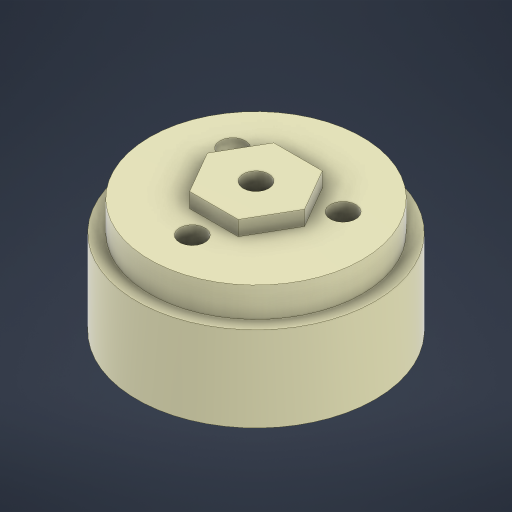
# Autodesk Inventor part: Shaft1_Joint1
Saved by Autodesk Inventor 2023 (Build 270158000, 158)
## iProperties
Created: 2023-02-21
Part Number: Shaft1_Joint1
Material: ABS Plastic
Document SubType Name: Modeling
Designer: dzw04
Density: 1.06 g/cm^3
Appearance: Smooth - Ash
Author: dzw04
Autodesk Inventor part; units mm, degrees
ref_plane "YZ Plane" through (0, 0, 0) normal (1, 0, 0) x (0, 1, 0)
ref_plane "XZ Plane" through (0, 0, 0) normal (0, 1, 0) x (-1, 0, 0)
ref_plane "XY Plane" through (0, 0, 0) normal (0, 0, 1) x (1, 0, 0)
sketch "Sketch1" plane through (0, 0, 0) normal (0, 1, 0) x (-1, 0, 0)
  circle A0 centre (0, 0) radius 14
  dimension "d0" = 28
  constraints: 1 centre point, 1 coincident
  measures "d0" diameter of A0
extrude "Extrusion1" add sketch "Sketch1" along normal blind 10
sketch "Sketch2" plane through (0, 10, 0) normal (0, 1, 0) x (1, 0, 0)
  circle A0 centre (0, 0) radius 12.5
  dimension "d3" = 25
  constraints: 1 centre point, 1 coincident
  measures "d3" diameter of A0
extrude "Extrusion2" add sketch "Sketch2" along normal blind 3.5
sketch "Sketch3" plane through (0, 0, 0) normal (0, -1, 0) x (1, 0, 0)
  circle A0 centre (0, 0) radius 7.5 construction
  circle A1 centre (0, 0) radius 1.5
  circle A2 centre (0, 7.5) radius 1.5
  circle A3 centre (-6.4952, 3.75) radius 1.5
  circle A4 centre (-6.4952, -3.75) radius 1.5
  circle A5 centre (0, -7.5) radius 1.5
  circle A6 centre (6.4952, -3.75) radius 1.5
  circle A7 centre (6.4952, 3.75) radius 1.5
  dimension "d6" = 15
  dimension "d7" = 3
  dimension "d8" = 3
  dimension "d11" = 360
  constraints: 7 centre point, 2 coincident, 1 vertical alignment, 15 other
  measures "d7" diameter of A1
  measures "d8" diameter of A2
extrude "Extrusion3" cut sketch "Sketch3" against normal through all contours A1 | A2 | A4 | A6
sketch "Sketch4" plane through (0, 0, 0) normal (0, -1, 0) x (1, 0, 0)
  circle A0 centre (0, 0) radius 7.5
  circle A1 centre (0, -7.5) radius 2.75
  circle A2 centre (0, 0) radius 7.5
  circle A3 centre (6.4952, -3.75) radius 2.75
  circle A4 centre (0, 0) radius 7.5
  circle A5 centre (6.4952, 3.75) radius 2.75
  circle A6 centre (0, 0) radius 7.5
  circle A7 centre (0, 7.5) radius 2.75
  circle A8 centre (0, 0) radius 7.5
  circle A9 centre (-6.4952, 3.75) radius 2.75
  circle A10 centre (0, 0) radius 7.5
  circle A11 centre (-6.4952, -3.75) radius 2.75
  dimension "d15" = 15
  dimension "d16" = 5.5
  dimension "d19" = 360
  constraints: 6 centre point, 2 vertical alignment, 1 coincident, 41 other
  measures "d16" diameter of A1
extrude "Extrusion4" cut sketch "Sketch4" against normal blind 6 contours A5 A0 | A0 A5 | A1 A0 | A0 A1 | A9 A0 | A0 A9
sketch "Sketch5" plane through (0, 13.5, 0) normal (0, 1, 0) x (1, 0, 0)
  line L0 (-2.8579, -4.95) -> (-5.7158, 0)
  line L1 (-5.7158, 0) -> (-2.8579, 4.95)
  line L2 (-2.8579, 4.95) -> (2.8579, 4.95)
  line L3 (2.8579, 4.95) -> (5.7158, 0)
  line L4 (5.7158, 0) -> (2.8579, -4.95)
  line L5 (2.8579, -4.95) -> (-2.8579, -4.95)
  circle A0 centre (0, 0) radius 1.5
  dimension "d23" = 9.9
  dimension "d29" = 3
  constraints: 12 end point, 2 coincident, 1 centre point, 1 horizontal, 13 other
  measures "d23" distance between parallel lines of L1 L4
  measures "d29" diameter of A0
extrude "Extrusion5" add sketch "Sketch5" along normal blind 1.75
body "Solid1"
